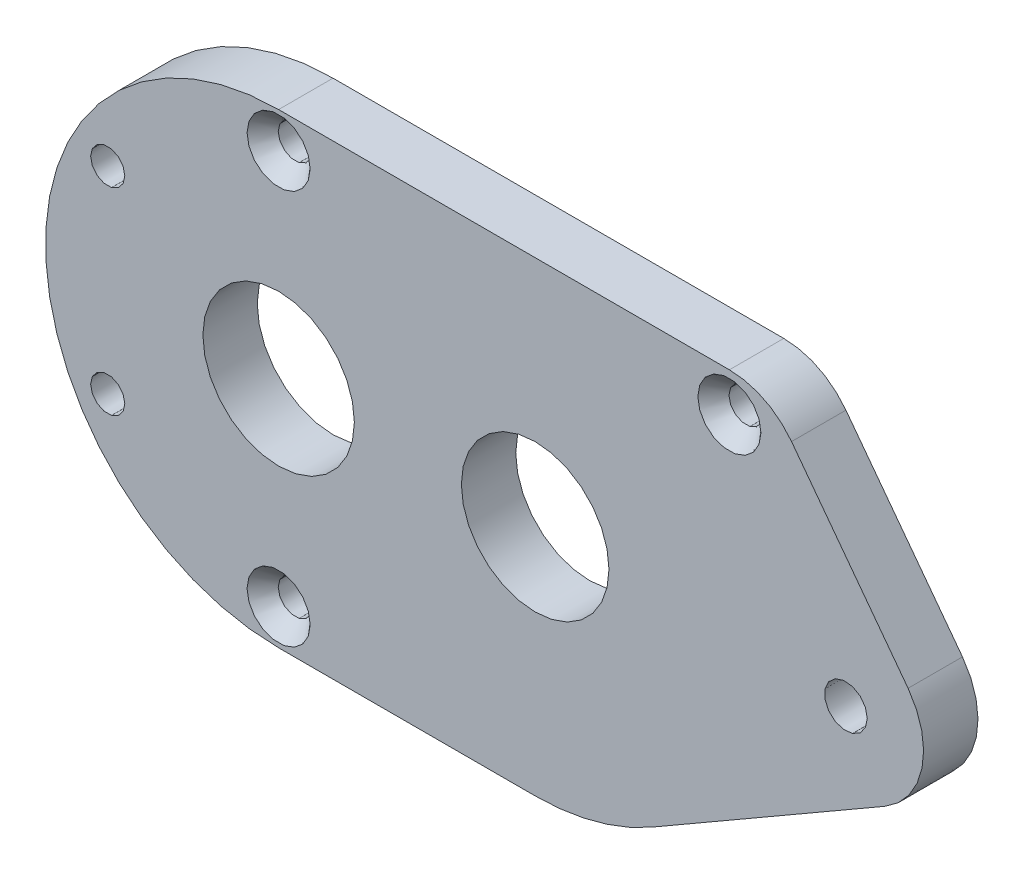
# Autodesk Inventor part: Outer Plate
Saved by Autodesk Inventor 2019.4 (Build 234330000, 330)
## iProperties
Created: 2020-01-01
Part Number: Outer Plate
Material: Aluminum 6061
Document SubType Name: Modeling
Designer: Mark
Mass: 92.7441 g
Surface Area: 132.725 cm^2
Volume: 34.3497 cm^3
Density: 2.7 g/cm^3
Appearance: Aluminum - Flat
Author: Mark
Autodesk Inventor part; units mm, degrees
ref_plane "YZ Plane" through (0, 0, 0) normal (1, 0, 0) x (0, 1, 0)
ref_plane "XZ Plane" through (0, 0, 0) normal (0, 1, 0) x (-1, 0, 0)
ref_plane "XY Plane" through (0, 0, 0) normal (0, 0, 1) x (1, 0, 0)
sketch "Sketch1" plane through (-26.51, 3.1066, 0) normal (0, 0, 1) x (1, 0, 0)
  circle A0 centre (0, 0) radius 7.62 construction
  circle A1 centre (0, 0) radius 9.75
  circle A2 centre (33.02, 0) radius 25.4 construction
  line L0 (0, 0) -> (7.62, 0)
  line L1 (0, 0) -> (7.62, 0) construction
  circle A3 centre (33.02, 0) radius 9.5
  line L2 (0, -30) -> (33.02, -30)
  line L3 (33.02, 30) -> (0, 30)
  arc A4 (33.02, -30) -> (63.02, 0) centre (33.02, 0) ccw
  arc A5 (0, 30) -> (0, -30) centre (0, 0) ccw
  circle A6 centre (0, 0) radius 25.4 construction
  line L4 (0, 25.4) -> (0, 0) construction
  line L5 (0, 25.4) -> (25.4, 25.4) construction
  circle A7 centre (0, 25.4) radius 2.2
  circle A8 centre (-21.997, 12.7) radius 2.2
  circle A9 centre (-21.997, -12.7) radius 2.2
  circle A10 centre (0, -25.4) radius 2.2
  circle A11 centre (21.997, -12.7) radius 2.2
  circle A12 centre (21.997, 12.7) radius 2.2
  line L6 (63.02, 0) -> (63.02, 30)
  line L7 (63.02, 30) -> (33.02, 30)
  circle A13 centre (58.02, 25) radius 2.2
  circle A14 centre (73.02, 0) radius 2.75
  circle A15 centre (73.02, 0) radius 10
  line L8 (81.02, 6) -> (63.02, 30)
  line L9 (78.02, -8.6603) -> (48.02, -25.9808)
  dimension "d13" = 50.8
  dimension "d21" = 15.24
  dimension "d20" = 19.5
  dimension "d18" = 50.8
  dimension "d17" = 7.62
  dimension "d25" = 0
  dimension "d19" = 33.02
  dimension "d16" = 19
  dimension "d14" = 30
  dimension "d15" = 60
  dimension "d26" = 25.4
  dimension "d27" = 90
  dimension "d12" = 4.4
  dimension "d2" = 360
  dimension "d11" = 30
  dimension "d9" = 30
  dimension "d10" = 90
  dimension "d6" = 4.4
  dimension "d8" = 5
  dimension "d7" = 5
  dimension "d4" = 5.5
  dimension "d5" = 10
  dimension "d3" = 20
  constraints: 20 end point, 15 centre point, 11 coincident, 7 point on circle, 4 horizontal, 4 tangent, 2 equal length, 2 parallel, 2 point on line, 1 equal radius, 1 perpendicular, 1 vertical alignment, 15 other
  measures "d21" diameter of A0
  measures "d20" diameter of A1
  measures "d18" diameter of A2
  measures "d17" distance of L0.start L0.end
  measures "d25" distance between parallel lines of L0 L1
  measures "d19" distance of A2.centre L0.start
  measures "d16" diameter of A3
  measures "d14" radius of A4
  measures "d15" distance between parallel lines of L3 L2
  measures "d26" distance of L4.start L4.end
  measures "d27" angle of L4 L5
  measures "d12" diameter of A7
  measures "d11" distance of L3.start L6.end
  measures "d9" distance of L6.start L6.end
  measures "d10" angle of L0 L6
  measures "d6" diameter of A13
  measures "d8" distance from line of L7 A13.centre
  measures "d7" distance from line of L6 A13.centre
  measures "d4" diameter of A14
  measures "d5" distance from line of L6 A14.centre
  measures "d3" diameter of A15
extrude "Extrusion1" add sketch "Sketch1" along normal blind 7 contours A5 L3 L7 L6 A4 L2 | A4 A15 L9 | L6 L8 A15 | A15 | A11 | A12
fillet "Fillet1" radius 10 1 edges at (36.51, 33.1066, 3.5)
sketch "Sketch2" plane through (-26.51, 3.1066, 7) normal (0, 0, 1) x (1, 0, 0)
  circle A0 centre (0, 25.4) radius 2.2 projected
  circle A1 centre (0, -25.4) radius 2.2 projected
  circle A2 centre (58.02, 25) radius 2.2 projected
  point P0 (26.51, -3.1066)
hole "Hole1" at (-26.51, 28.5066, 7) at (31.51, 28.1066, 7) at (-26.51, -22.2934, 7) direction (0, 0, -1) diameter 4.4 depth 7 countersink diameter 8.13 countersink angle 82
body "Solid1"
